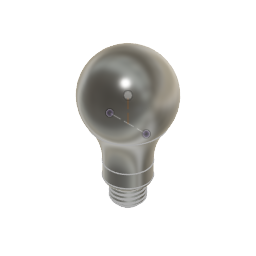
Day 9 - Light Bulb (Autodesk Fusion 360 design; units mm, degrees)
part number: 2025-06-17-11-40-34-205
Autodesk Fusion 360 part; units mm, degrees
cylinder "CylinderPrimitive1" add diameter 30 height 40 placed x (1, 0, 0) y (0, 1, 0) z (0, 0, 1) at (0, 0, 0) makes body 1
sketch "Sketch2" plane through (0, 0, 0) normal (0, 1, 0) x (1, 0, 0)
  line L0 (-15, -40) -> (-13.5737, -40)
  line L1 (-13.5737, -40) -> (15, -40) construction
  line L2 (0, -40) -> (0, -60) construction
  point P0 (-15, -40)
  point P1 (15, -40)
  dimension "d4" = 20
  constraint coincident P0 L0.start
  constraint horizontal L0
  constraint coincident P1 L1.end
  constraint parallel L0 L1
  constraint coincident L1 L2.start
  constraint perpendicular L1 L2
  measures "d4" distance of L2.start L2.end
sphere "SpherePrimitive1" add diameter 61 placed x (1, 0, 0) y (0, 0, -1) z (0, 1, 0) at (0, 0, 60) bodies 1
fillet "Fillet1" radius 45 1 edges at (-13.9849, 5.4242, 33.4435) on bodies 1
fillet "Fillet1" radius 4 1 edges at (-13.9849, 5.4242, 0) on bodies 1
cylinder "CylinderPrimitive2" add diameter 22 height 15 placed x (0, 1, 0) y (1, 0, 0) z (0, 0, -1) at (0, 0, 0) separate body makes body 2
thread "Thread1" "ANSI Metric M Profile 22.0 M22x3 M22x3 6g" major diameter 21.7645 minor diameter 18.3374 pitch 3 angle 60 modelled right hand crest width 0.4298 on face at (-1.0952, 10.9453, -5) from (0, 0, 0) to (0, 0, -12) crest through (0, 10.8823, 0.75) on bodies 2
chamfer "Chamfer1" distance 4 angle 45 1 edges at (-3.9352, -10.1458, -15) measured on face at (-0.3528, 2.3404, -15) on bodies 2
fillet "Fillet2" radius 2 1 faces at (0.2969, -0.1714, -15) on bodies 2
cylinder "CylinderPrimitive3" add diameter 12.108 height 2 placed x (0, 1, 0) y (1, 0, 0) z (0, 0, -1) at (0, 0, -15) separate body makes body 3
chamfer "Chamfer2" distance 2 angle 45 1 edges at (-2.1892, -5.6443, -17) measured on face at (-1.2257, 0.481, -17) on bodies 3
